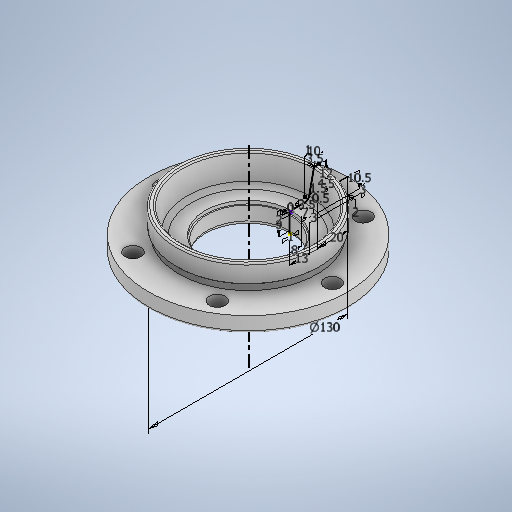
# Autodesk Inventor part: 05_Nap_o_thung
Saved by Autodesk Inventor 2025.2 (Build 292293000, 293)
## iProperties
Created: 2024-11-27
Part Number: 05_Nap_o_thung
Material: Generic
Document SubType Name: Modeling
Designer: hongquan
Density: 1 g/cm^3
Appearance: Default
Author: hongquan
Autodesk Inventor part; units mm, degrees
ref_plane "YZ Plane" through (0, 0, 0) normal (1, 0, 0) x (0, 1, 0)
ref_plane "XZ Plane" through (0, 0, 0) normal (0, 1, 0) x (-1, 0, 0)
ref_plane "XY Plane" through (0, 0, 0) normal (0, 0, 1) x (1, 0, 0)
sketch "Sketch1" plane through (0, 0, 0) normal (1, 0, 0) x (0, 1, 0)
  line L0 (0, 0) -> (0, -13)
  line L1 (0, -13) -> (0, -13)
  line L2 (3, -16.8284) -> (3, -36)
  line L3 (5, -38) -> (13.5, -38)
  line L4 (13.5, -38) -> (13.5, -18)
  line L5 (13.5, -18) -> (17.5, -18)
  arc A0 (3, -36) -> (5, -38) centre (5, -36) ccw
  line L6 (0, -13) -> (2.4142, -15.4142)
  arc A1 (3, -16.8284) -> (2.4142, -15.4142) centre (1, -16.8284) ccw
  line L7 (13, 0) -> (0, 0)
  line L8 (64.2413, 27) -> (-63.4715, 27)
  line L9 (11, 0) -> (2, 0) construction
  line L10 (11, 0) -> (13, 0)
  line L11 (2, 0) -> (0, 0)
  line L12 (11, 0) -> (10, -8)
  line L13 (10, -8) -> (3, -8)
  line L14 (3, -8) -> (2, 0)
  line L15 (6.5, 0) -> (6.5, -8) construction
  line L16 (13, -1) -> (10.875, -1)
  line L17 (2.125, -1) -> (0, -1)
  line L18 (18, -18.5) -> (18, -19)
  line L19 (18.5, -19.5) -> (29, -19.5)
  line L20 (30, -18.5) -> (30, -16.8065)
  line L21 (0, -13) -> (13, -13) construction
  line L22 (13, -9.5) -> (0, -9.5) construction
  line L23 (29.2118, -15.8292) -> (0, -9.5) construction
  line L24 (13, 0) -> (13, -9.8971)
  line L25 (30, -16) -> (15.3647, -12.829)
  arc A2 (13, -9.8971) -> (15.3647, -12.829) centre (16, -9.8971) ccw
  arc A3 (30, -16.8065) -> (29.2118, -15.8292) centre (29, -16.8065) ccw
  arc A4 (29, -19.5) -> (30, -18.5) centre (29, -18.5) ccw
  arc A5 (18, -19) -> (18.5, -19.5) centre (18.5, -19) ccw
  arc A6 (18, -18.5) -> (17.5, -18) centre (17.5, -18.5) ccw
  point P0 (3, -13)
  point P1 (3, -38)
  point P2 (13, -18)
  point P3 (18, -18)
  point P4 (11.9375, -1)
  point P5 (18, -19.5)
  point P6 (30, -19.5)
  point P7 (13, -12.3167)
  point P8 (29.2118, -15.8292)
  dimension "d1" = 10.5
  dimension "d2" = 13
  dimension "d3" = 3
  dimension "d5" = 20
  dimension "d16" = 2
  dimension "d20" = 130
  dimension "d36" = 7
  dimension "d37" = 2
  dimension "d38" = 0
  dimension "d39" = 8
  dimension "d40" = 1
  dimension "d41" = 1
  dimension "d43" = 1.5
  dimension "d44" = 4.5
  dimension "d45" = 12
  dimension "d46" = 3.5
  dimension "d47" = 3.5
  dimension "d48" = 10
  dimension "d49" = 3
  dimension "d50" = 1
  dimension "d51" = 0.5
  dimension "d52" = 9
  constraints: 52 end point, 21 point on line, 14 point on circle, 14 tangent, 10 perpendicular, 7 centre point, 7 horizontal, 4 vertical, 3 midpoint, 2 collinear, 2 equal radius, 1 other
  measures "d1" distance of point (3, -38) L3.end
  measures "d2" distance of L0.start L0.end
  measures "d3" distance of L0.end point (3, -13)
  measures "d5" distance of L3.end L4.end
  measures "d16" radius of A0
  measures "d20" diameter of L3 L8
  measures "d36" distance of L12.end L13.end
  measures "d37" distance of L9.start L10.end
  measures "d38" distance between parallel lines of L7 L9
  measures "d39" distance of L15.start L15.end
  measures "d40" distance from line of L7 point (11.937, -1)
  measures "d41" distance between parallel lines of L7 L17
  measures "d43" distance of point (18, -18) point (18, -19.5)
  measures "d44" distance of L4.end point (18, -18)
  measures "d45" distance of point (18, -19.5) point (30, -19.5)
  measures "d46" distance of point (30, -19.5) L25.start
  measures "d47" distance of L21.end L22.start
  measures "d48" distance from line of L19 L22.start
  measures "d49" radius of A2
  measures "d50" radius of A3
  measures "d51" radius of A5
  measures "d52" distance of L9.start L9.end
revolve "Revolution1" add sketch "Sketch1" angle 360 about axis through (0, 64.2413, 27) along (0, -1, 0) contours L17 L14 L13 L12 L16 L24 A2 L25 A3 L20 A4 L19 A5 L18 A6 L5 L4 L3 A0 L2 A1 L6 L0 | L7 L12 L13 L14
sketch "Sketch3" plane through (0, 3, 27) normal (0, -1, 0) x (1, 0, 0)
  circle A0 centre (0, 0) radius 55
  circle A1 centre (0, 0) radius 63 projected
  circle A2 centre (-55, 0) radius 5.25
  line L0 (72.7764, 0) -> (-106.6321, 0) construction
  point P0 (0, -27)
  dimension "d53" = 110
  dimension "d55" = 10.5
  constraints: 2 end point, 2 horizontal, 1 centre point, 1 coincident, 1 horizontal alignment, 1 point on line, 3 other
  measures "d55" diameter of A2
hole "Hole2" at (-55, 3, 27) direction (0, 1, 0) diameter 10.5 end through all
chamfer "Chamfer2" distance 0.5 angle 45 1 edges at (-55, 3, 32.25)
pattern_circular "Circular Pattern2" count 6 over 360 about axis through (0, 9.25, 27) along (0, -1, 0) of "Hole2"
sketch "Sketch4" plane through (0, 0, 27) normal (0, -1, 0) x (1, 0, 0)
  point P0 (0, -27)
body "Solid1"
